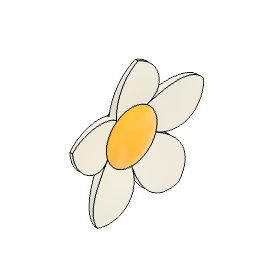
flower (Autodesk Fusion 360 design; units mm, degrees)
part number: 2025-09-15-23-24-38-197
Autodesk Fusion 360 part; units mm, degrees
sketch "Sketch1" plane through (0, 0, 0) normal (0, 1, 0) x (1, 0, 0)
  line L0 (0, 0) -> (-32, 0)
  line L1 (-32, 0) -> (-32, -26)
  line L2 (-32, -26) -> (-22, -36)
  line L3 (-22, -36) -> (-10.6827, -36)
  arc A0 (-10.6827, -36) -> (0, 0) centre (-66, 0) ccw
  arc A1 (-1.5763, -98) -> (-10.6827, -36) centre (-98, -80.4938) ccw
  line L4 (0, 0) -> (0, -90) construction
  arc A2 (-5.5763, -98) -> (-22, -36) centre (-117.5209, -94.4787) ccw
  line L5 (-1.5763, -98) -> (-5.5763, -98)
  dimension "d1" = 66
  dimension "d2" = 32
  dimension "d3" = 36
  dimension "d4" = 135
  dimension "d5" = 10
  dimension "d6" = 98
  dimension "d7" = 98
  dimension "d8" = 112
  dimension "d9" = 4
  constraint coincident L0.start A0.end
  constraint horizontal L0
  constraint perpendicular L0 L1
  constraint perpendicular L1 L3
  constraint horizontal L0.end A0.centre
  constraint tangent A0 L4
  constraint perpendicular L0 L4
  constraint tangent A1 L4
  constraint horizontal L5
  measures "d1" radius of A0
  measures "d2" distance of L0.start L0.end
  measures "d3" distance of L0 L2.end
  measures "d4" angle of L1 L2
  measures "d5" horizontal distance of L1.end L2.end
  measures "d6" distance of L0 A1.start
  measures "d7" radius of A1
  measures "d8" radius of A2
  measures "d9" horizontal distance of A1.start A2.start
revolve "Revolve1" add sketch "Sketch1" angle 360 about axis through (0, 0, 0) along (-1, 0, 0) contours L0 L1 L2 L3 A0 makes body 1
revolve "Revolve2" add sketch "Sketch1" angle 360 about axis through (0, 0, 0) along (-1, 0, 0) separate body contours L3 A1 A2 L5 makes body 2
sketch "Sketch3" plane through (0, 0, 0) normal (1, 0, 0) x (0, 1, 0)
  circle A0 centre (0, 0) radius 98
  circle A1 centre (0, 0) radius 36
  line L0 (0, 0) -> (-21.1603, 29.1246)
  line L1 (0, 0) -> (0, 90)
  arc A2 (0, 98) -> (-21.1603, 29.1246) centre (15.2968, 55.6122) ccw
  arc A3 (21.1603, 29.1246) -> (0, 98) centre (-15.2968, 55.6122) ccw
  point P0 (0, 98)
  dimension "d12" = 36
  constraint coincident A0.centre A1.centre
  constraint coincident A1 L0.end
  constraint coincident A0 P0
  constraint tangent L0 A2
  constraint coincident P0 A2.start
  constraint symmetric L0.end L1 A3.start
  constraint symmetric L1 P0 A2.start
  constraint symmetric L1 A2 A3
  measures "d12" angle of L0 L1
extrude "Extrude1" cut sketch "Sketch3" against normal through all contours A1 A2 A3 keep common part bodies 2
pattern_circular "C-Pattern1" count 5 over 360 about axis through (-10.6827, 0, 0) along (-1, 0, 0) of bodies 2 makes body 3 at (-6.2405, 77.3432, 26.642) makes body 4 at (-17.9931, 4.2624, -42.9038) makes body 5 at (-17.9931, -39.4868, -17.3118) makes body 6 at (-6.2405, -77.3432, 26.642)
combine "Combine1" operation add target body 6 tool bodies 3 2 5 4 1
